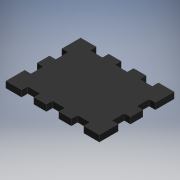
# Autodesk Inventor part: left
Saved by Autodesk Inventor 2019 (Build 230136000, 136)
## iProperties
Created: 2018-06-06
Part Number: left
Material: PBT Plastic Black
Document SubType Name: Modeling
Designer: stra92745
Density: 1.31 g/cm^3
Appearance: Smooth - White
Author: stra92745
Autodesk Inventor part; units mm, degrees
ref_plane "YZ Plane" through (0, 0, 0) normal (1, 0, 0) x (0, 1, 0)
ref_plane "XZ Plane" through (0, 0, 0) normal (0, 1, 0) x (-1, 0, 0)
ref_plane "XY Plane" through (0, 0, 0) normal (0, 0, 1) x (1, 0, 0)
sketch "Sketch1" plane through (0, 0, 0) normal (0, 1, 0) x (-1, 0, 0)
  line L0 (0, 0) -> (-60, 0)
  line L1 (-60, 0) -> (-60, -48)
  line L2 (-60, -48) -> (0, -48)
  line L3 (0, -48) -> (0, 0)
  dimension "d0" = 60
  dimension "d1" = 48
  constraints: 8 end point, 2 parallel, 1 horizontal, 1 perpendicular
  measures "d0" distance of L2.end L1.end
  measures "d1" distance of L1.end L0.end
extrude "Extrusion1" add sketch "Sketch1" along normal blind 4
sketch "Sketch2" plane through (0, 4, 0) normal (0, 1, 0) x (1, 0, 0)
  line L0 (0, 0) -> (60, 0) construction
  line L1 (60, 0) -> (60, 48) construction
  line L2 (60, 48) -> (0, 48) construction
  line L3 (0, 48) -> (0, 0) construction
  line L4 (4, 44) -> (56, 44) construction
  line L5 (56, 44) -> (56, 4) construction
  line L6 (56, 4) -> (4, 4) construction
  line L7 (4, 4) -> (4, 44) construction
  line L8 (60, 48) -> (0, 48) construction
  line L9 (30, 48) -> (30, 0) construction
  line L10 (0, 0) -> (60, 0) construction
  line L11 (0, 48) -> (0, 0) construction
  line L12 (0, 24) -> (60, 24) construction
  line L13 (60, 0) -> (60, 48) construction
  line L14 (0, 28) -> (4, 28)
  line L15 (0, 36) -> (4, 36)
  line L16 (10, 48) -> (10, 44)
  line L17 (10, 44) -> (18, 44)
  line L18 (18, 44) -> (18, 48)
  line L19 (18, 48) -> (10, 48)
  line L20 (26, 48) -> (26, 44)
  line L21 (26, 44) -> (30, 44)
  line L22 (26, 48) -> (30, 48)
  line L23 (0, 36) -> (0, 28)
  line L24 (4, 28) -> (4, 36)
  line L25 (60, 28) -> (56, 28)
  line L26 (60, 36) -> (56, 36)
  line L27 (50, 48) -> (50, 44)
  line L28 (50, 44) -> (42, 44)
  line L29 (42, 44) -> (42, 48)
  line L30 (42, 48) -> (50, 48)
  line L31 (34, 48) -> (34, 44)
  line L32 (34, 44) -> (30, 44)
  line L33 (34, 48) -> (30, 48)
  line L34 (60, 36) -> (60, 28)
  line L35 (56, 28) -> (56, 36)
  line L36 (60, 0) -> (0, 0) construction
  line L37 (4, 4) -> (56, 4) construction
  line L38 (60, 0) -> (0, 0) construction
  line L39 (0, 20) -> (4, 20)
  line L40 (0, 12) -> (4, 12)
  line L41 (10, 0) -> (10, 4)
  line L42 (10, 4) -> (18, 4)
  line L43 (18, 4) -> (18, 0)
  line L44 (18, 0) -> (10, 0)
  line L45 (26, 0) -> (26, 4)
  line L46 (26, 4) -> (30, 4)
  line L47 (26, 0) -> (30, 0)
  line L48 (0, 12) -> (0, 20)
  line L49 (4, 20) -> (4, 12)
  line L50 (34, 0) -> (34, 4)
  line L51 (34, 4) -> (30, 4)
  line L52 (34, 0) -> (30, 0)
  line L53 (42, 4) -> (42, 0)
  line L54 (50, 4) -> (42, 4)
  line L55 (42, 0) -> (50, 0)
  line L56 (50, 0) -> (50, 4)
  line L57 (56, 20) -> (56, 12)
  line L58 (60, 12) -> (56, 12)
  line L59 (60, 12) -> (60, 20)
  line L60 (60, 20) -> (56, 20)
  dimension "d4" = 4
  dimension "d7" = 8
  dimension "d8" = 8
  dimension "d9" = 4
  dimension "d10" = 8
  dimension "d11" = 4
  constraints: 106 end point, 31 symmetric about line, 16 point on line, 6 midpoint, 4 perpendicular, 3 collinear, 1 horizontal, 1 vertical, 3 other
  measures "d4" distance between parallel lines of L2 L4
  measures "d7" distance between parallel lines of L14 L15
  measures "d8" distance of L16.end L17.end
  measures "d9" distance of L20.end L21.end
  measures "d10" distance between parallel lines of L18 L20
  measures "d11" distance between parallel lines of L12 L14
extrude "Extrusion2" cut sketch "Sketch2" against normal up to surface (4 mm away)
body "Solid1"
